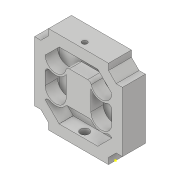
# Autodesk Inventor part: 20_Cube_Inser_Flexuremanipulator_zonly_translation_v3
Saved by Autodesk Inventor 2019.4 (Build 234330000, 330)
## iProperties
Created: 2019-07-01
Part Number: 20_Cube_Inser_Flexuremanipulator_zonly_translation_v3
Material: Generic
Document SubType Name: Modeling
Designer: diederichbenedict
Density: 1 g/cm^3
Appearance: Default
Author: diederichbenedict
Autodesk Inventor part; units mm, degrees
ref_plane "YZ Plane" through (0, 0, 0) normal (1, 0, 0) x (0, 1, 0)
ref_plane "XZ Plane" through (0, 0, 0) normal (0, 1, 0) x (-1, 0, 0)
ref_plane "Work Plane1" through (0, 0, 10) normal (0, 0, 1) x (1, 0, 0)
sketch "Sketch1" plane through (0, 0, 10) normal (0, 0, 1) x (1, 0, 0)
  line L0 (-4.0299, -0.3538) -> (-2.2322, 1.4439) construction
  arc A0 (-1.4439, 2.2322) -> (-2.2322, 1.4439) centre (-0.9299, 0.9299) ccw construction
  line L1 (-1.4439, 2.2322) -> (0.3538, 4.0299) construction
  line L2 (-37.8299, 42.8299) -> (-37.8299, 37.8299) construction
  line L3 (-37.8299, 37.8299) -> (-42.9208, 37.8299) construction
  line L4 (-37.8299, 42.2137) -> (-37.8299, 45.8299) construction
  line L5 (-37.8299, 45.8299) -> (-4.0299, 45.8299) construction
  line L6 (-4.0299, 45.8299) -> (-4.0299, 42.2137) construction
  line L7 (-4.0299, 4.0299) -> (0.3538, 4.0299) projected
  circle A1 centre (-20.9299, 20.9299) radius 17.5 projected
  line L8 (-20.9299, 58.9723) -> (17.1124, 20.9299) construction
  line L9 (17.1124, 20.9299) -> (-20.9299, -17.1124) construction
  line L10 (-20.9299, -17.1124) -> (-58.9723, 20.9299) construction
  line L11 (-58.9723, 20.9299) -> (-20.9299, 58.9723) construction
  line L12 (-20.9299, 58.9723) -> (-20.9299, -17.1124) construction
  line L13 (17.1124, 20.9299) -> (-58.9723, 20.9299) construction
  line L14 (-20.9299, 58.9723) -> (32.8701, 58.9723) construction
  line L15 (-43.4299, 43.4299) -> (1.5701, 43.4299) construction
  line L16 (1.5701, 43.4299) -> (1.5701, -1.5701) construction
  line L17 (1.5701, -1.5701) -> (-43.4299, -1.5701) construction
  line L18 (-43.4299, -1.5701) -> (-43.4299, 43.4299) construction
  line L19 (-43.4299, 43.4299) -> (1.5701, -1.5701) construction
  line L20 (1.5701, 43.4299) -> (-43.4299, -1.5701) construction
  line L21 (-43.4299, 5.3876) -> (-43.4299, 36.4723)
  line L22 (-43.4299, 36.4723) -> (-36.4723, 43.4299)
  line L23 (-36.4723, 43.4299) -> (-5.3876, 43.4299)
  line L24 (-5.3876, 43.4299) -> (1.5701, 36.4723)
  line L25 (1.5701, 36.4723) -> (1.5701, 5.3876)
  line L26 (1.5701, 5.3876) -> (-5.3876, -1.5701)
  line L27 (-5.3876, -1.5701) -> (-36.4723, -1.5701)
  line L28 (-36.4723, -1.5701) -> (-43.4299, 5.3876)
  line L29 (-4.0299, 42.2137) -> (-37.8299, 42.2137) projected
  line L30 (-4.0299, -0.3538) -> (-4.0299, 4.0299) projected
  circle A2 centre (-20.9299, 20.9299) radius 1.5
  line L31 (-10.9299, 10.9299) -> (-30.9299, 10.9299) construction
  line L32 (-30.9299, 10.9299) -> (-30.9299, 30.9299) construction
  line L33 (-30.9299, 30.9299) -> (-10.9299, 30.9299) construction
  line L34 (-10.9299, 30.9299) -> (-10.9299, 10.9299) construction
  line L35 (-10.9299, 10.9299) -> (-30.9299, 30.9299) construction
  line L36 (-30.9299, 10.9299) -> (-10.9299, 30.9299) construction
  circle A3 centre (-30.9299, 30.9299) radius 1.4
  circle A4 centre (-30.9299, 10.9299) radius 1.4
  circle A5 centre (-10.9299, 10.9299) radius 1.4
  line L37 (-45.8299, 37.8299) -> (-42.0723, 37.8299) construction
  line L38 (-42.1723, 37.7299) -> (-45.8299, 37.7299)
  line L39 (-45.8299, 37.7299) -> (-45.8299, 4.1299)
  line L40 (-45.8299, 4.1299) -> (-42.1723, 4.1299)
  line L41 (-42.1723, 4.1299) -> (-42.1723, 37.7299)
  line L42 (-45.8299, 4.0299) -> (-42.0723, 4.0299) construction
  line L43 (-45.8299, 37.8299) -> (-42.0723, 37.8299) projected
  line L44 (-37.7299, 45.8299) -> (-4.1299, 45.8299)
  line L45 (-4.1299, 45.8299) -> (-4.1299, 42.1723)
  line L46 (-4.1299, 42.1723) -> (-37.7299, 42.1723)
  line L47 (-37.7299, 42.1723) -> (-37.7299, 45.8299)
  line L48 (0.4701, 37.8299) -> (0.4701, 4.0299) construction
  line L49 (0.4701, 4.0299) -> (3.9701, 4.0299) construction
  line L50 (3.9701, 37.8299) -> (3.9701, 4.0299) construction
  line L51 (0.4701, 37.8299) -> (3.9701, 37.8299) construction
  line L52 (-45.8299, -3.9701) -> (-4.0299, -3.9701) construction
  line L53 (0.3124, 37.7299) -> (3.9701, 37.7299)
  line L54 (3.9701, 37.7299) -> (3.9701, 4.1299)
  line L55 (3.9701, 4.1299) -> (0.3124, 4.1299)
  line L56 (0.3124, 4.1299) -> (0.3124, 37.7299)
  line L57 (-4.1713, -0.3538) -> (-37.7299, -0.3538)
  line L58 (-37.7299, -0.3538) -> (-37.7299, -3.9701)
  line L59 (-37.7299, -3.9701) -> (-4.1713, -3.9701)
  line L60 (-4.1713, -3.9701) -> (-4.1713, -0.3538)
  point P0 (-37.8299, 4.0299)
  dimension "d18" = 53.8
  dimension "d19" = 45
  dimension "d20" = 53.8
  dimension "d21" = 45
  dimension "d22" = 45
  dimension "d30" = 20
  dimension "d31" = 20
  dimension "d32" = 2.8
  dimension "d33" = 2.8
  dimension "d34" = 2.8
  dimension "d35" = 3
  dimension "d36" = 0.1
  dimension "d37" = 0.1
  dimension "d38" = 0.1
  dimension "d39" = 0.1
  constraints: 86 end point, 21 point on line, 14 parallel, 8 perpendicular, 7 horizontal, 7 midpoint, 4 centre point, 4 coincident, 1 equal length
  measures "d18" distance of L8.start L8.end
  measures "d19" angle of L8 L14
  measures "d20" distance of L8.end L9.end
  measures "d21" distance of L16.end L17.end
  measures "d22" distance of L15.end L16.end
  measures "d30" distance of L32.end L33.end
  measures "d31" distance of L31.end L32.end
  measures "d32" diameter of A3
  measures "d33" diameter of A4
  measures "d34" diameter of A5
  measures "d35" diameter of A2
  measures "d36" distance between parallel lines of L38 L43
  measures "d37" distance between parallel lines of L40 L42
  measures "d38" distance between parallel lines of L45 L6
  measures "d39" distance between parallel lines of L4 L47
extrude "Extrusion1" add sketch "Sketch1" along normal blind 5 contours L30 L26 L57 L28 L41 L22 L46 L24 L56 L7 | L7 L26 L30 | L56 L24 L25 L26 | L26 L25 L24 L53 L54 L55 | L60 L59 L58 L57 L28 L27 L26 | L26 L27 L28 L57 | L46 L22 L29 L24 | L24 L29 L45 | L40 L39 L38 L22 L21 L28 | L28 L21 L22 L41 | L29 L22 L23 L24 | L24 L23 L22 L29 L47 L44 L45 | L47 L29 L22 | A1 | A2 | A3 | A4 | A5
sketch "Skizze4" plane through (0, 0, 15) normal (0, 0, 1) x (1, 0, 0)
  line L0 (-37.7299, 42.1723) -> (-42.1723, 37.7299) projected
  line L1 (-42.1723, 37.7299) -> (-45.8299, 37.7299) projected
  line L2 (-45.8299, 37.7299) -> (-45.8299, 4.1299) construction
  line L3 (-45.8299, 4.1299) -> (-42.1723, 4.1299) projected
  line L4 (-42.1723, 4.1299) -> (-37.6885, -0.3538) projected
  line L5 (-37.6885, -0.3538) -> (-37.7299, -0.3538) projected
  line L6 (-37.7299, -0.3538) -> (-37.7299, -3.9701) projected
  line L7 (-37.7299, -3.9701) -> (-4.1713, -3.9701) construction
  line L8 (-4.1713, -3.9701) -> (-4.1713, -0.3538) projected
  line L9 (-4.1713, -0.3538) -> (0.3124, 4.1299) projected
  line L10 (0.3124, 4.1299) -> (3.9701, 4.1299) projected
  line L11 (3.9701, 4.1299) -> (3.9701, 37.7299) construction
  line L12 (3.9701, 37.7299) -> (0.3124, 37.7299) projected
  line L13 (0.3124, 37.7299) -> (-4.1299, 42.1723) projected
  line L14 (-4.1299, 42.1723) -> (-4.1299, 45.8299) projected
  line L15 (-4.1299, 45.8299) -> (-37.7299, 45.8299) construction
  line L16 (-37.7299, 45.8299) -> (-37.7299, 42.1723) projected
  line L17 (-37.9299, 46.0299) -> (-3.9299, 46.0299) construction
  line L18 (-3.9299, 46.0299) -> (-3.9299, 42.2551)
  line L19 (-3.9299, 42.2551) -> (0.3953, 37.9299)
  line L20 (0.3953, 37.9299) -> (4.1701, 37.9299)
  line L21 (4.1701, 37.9299) -> (4.1701, 3.9299) construction
  line L22 (4.1701, 3.9299) -> (0.3953, 3.9299)
  line L23 (0.3953, 3.9299) -> (-3.9713, -0.4367)
  line L24 (-3.9713, -0.4367) -> (-3.9713, -4.1701)
  line L25 (-3.9713, -4.1701) -> (-37.9299, -4.1701) construction
  line L26 (-37.9299, -4.1701) -> (-37.9299, -0.3953)
  line L27 (-37.9299, -0.3953) -> (-42.2551, 3.9299)
  line L28 (-42.2551, 3.9299) -> (-46.0299, 3.9299)
  line L29 (-46.0299, 3.9299) -> (-46.0299, 37.9299) construction
  line L30 (-46.0299, 37.9299) -> (-42.2551, 37.9299)
  line L31 (-42.2551, 37.9299) -> (-37.9299, 42.2551)
  line L32 (-37.9299, 42.2551) -> (-37.9299, 46.0299)
  line L33 (-45.8299, 37.7299) -> (-45.8299, 37.9299)
  line L34 (-4.1299, 45.8299) -> (-37.7299, 45.8299) projected
  line L35 (-37.7299, 45.8299) -> (-37.9299, 45.8299)
  line L36 (-4.1299, 45.8299) -> (-3.9299, 45.8299)
  line L37 (3.9701, 37.7299) -> (3.9701, 37.9299)
  line L38 (3.9701, 4.1299) -> (3.9701, 37.7299) projected
  line L39 (3.9701, 4.1299) -> (3.9701, 3.9299)
  line L40 (-4.1713, -3.9701) -> (-3.9713, -3.9701)
  line L41 (-37.7299, -3.9701) -> (-37.9299, -3.9701)
  line L42 (-45.8299, 4.1299) -> (-45.8299, 3.9299)
  point P0 (0, 0)
  dimension "d40" = 0.2
  constraints: 48 end point, 12 point on line, 4 perpendicular, 15 other
  measures "d40" distance between parallel lines of L15 L17
extrude "IM_offset" add sketch "Skizze4" against normal up to surface (5 mm away)
sketch "Sketch5" plane through (0, 0, 15) normal (0, 0, 1) x (1, 0, 0)
  line L0 (-3.9299, 45.8299) -> (-37.9299, 45.8299) projected
  line L1 (-37.9299, 45.8299) -> (-37.9299, 42.2551) projected
  line L2 (-37.9299, 42.2551) -> (-42.2551, 37.9299) projected
  line L3 (-42.2551, 37.9299) -> (-45.8299, 37.9299) projected
  line L4 (-45.8299, 37.9299) -> (-45.8299, 3.9299) projected
  line L5 (-42.2551, 3.9299) -> (-45.8299, 3.9299) projected
  line L6 (-37.9299, -0.3953) -> (-42.2551, 3.9299) projected
  line L7 (-37.9299, -3.9701) -> (-37.9299, -0.3953) projected
  line L8 (-3.9713, -3.9701) -> (-37.9299, -3.9701) projected
  line L9 (-3.9713, -3.9701) -> (-3.9713, -0.4367) projected
  line L10 (-3.9713, -0.4367) -> (0.3953, 3.9299) projected
  line L11 (0.3953, 3.9299) -> (3.9701, 3.9299) projected
  line L12 (3.9701, 3.9299) -> (3.9701, 37.9299) projected
  line L13 (3.9701, 37.9299) -> (0.3953, 37.9299) projected
  line L14 (0.3953, 37.9299) -> (-3.9299, 42.2551) projected
  line L15 (-3.9299, 42.2551) -> (-3.9299, 45.8299) projected
  line L16 (-2.0299, 31.9299) -> (-2.0299, 9.9299)
  line L17 (-2.0299, 9.9299) -> (-2.09, 9.9299)
  line L18 (-2.09, 9.9299) -> (-9.9713, 2.0486)
  line L19 (-9.9713, 2.0486) -> (-9.9713, 2.0299)
  line L20 (-9.9713, 2.0299) -> (-31.9299, 2.0299)
  line L21 (-31.9299, 2.0299) -> (-31.9299, 2.09)
  line L22 (-31.9299, 2.09) -> (-39.7698, 9.9299)
  line L23 (-39.7698, 9.9299) -> (-39.8299, 9.9299)
  line L24 (-39.8299, 9.9299) -> (-39.8299, 31.9299)
  line L25 (-39.8299, 31.9299) -> (-39.7698, 31.9299)
  line L26 (-39.7698, 31.9299) -> (-31.9299, 39.7698)
  line L27 (-31.9299, 39.7698) -> (-31.9299, 39.8299)
  line L28 (-31.9299, 39.8299) -> (-9.9299, 39.8299)
  line L29 (-9.9299, 39.8299) -> (-9.9299, 39.7698)
  line L30 (-9.9299, 39.7698) -> (-2.09, 31.9299)
  line L31 (-2.09, 31.9299) -> (-2.0299, 31.9299)
  dimension "d46" = 6
  constraints: 32 end point, 15 other
  measures "d46" distance between parallel lines of L12 L16
extrude "Extrusion5" add sketch "Sketch5" along normal blind 8
sketch "Sketch6" plane through (0, 0, 23) normal (0, 0, 1) x (1, 0, 0)
  point P0 (0, 0)
sketch "Sketch7" plane through (0, 0, 23) normal (0, 0, 1) x (1, 0, 0)
  line L0 (-2.0299, 9.9299) -> (-2.09, 9.9299) projected
  line L1 (-2.09, 9.9299) -> (-9.9713, 2.0486) projected
  line L2 (-9.9713, 2.0486) -> (-9.9713, 2.0299) projected
  line L3 (-9.9713, 2.0299) -> (-31.9299, 2.0299) projected
  line L4 (-31.9299, 2.0299) -> (-31.9299, 2.09) projected
  line L5 (-31.9299, 2.09) -> (-39.7698, 9.9299) projected
  line L6 (-39.7698, 9.9299) -> (-39.8299, 9.9299) projected
  line L7 (-39.8299, 9.9299) -> (-39.8299, 31.9299) projected
  line L8 (-39.8299, 31.9299) -> (-39.7698, 31.9299) projected
  line L9 (-39.7698, 31.9299) -> (-31.9299, 39.7698) projected
  line L10 (-31.9299, 39.7698) -> (-31.9299, 39.8299) projected
  line L11 (-31.9299, 39.8299) -> (-9.9299, 39.8299) projected
  line L12 (-9.9299, 39.8299) -> (-9.9299, 39.7698) projected
  line L13 (-9.9299, 39.7698) -> (-2.09, 31.9299) projected
  line L14 (-2.09, 31.9299) -> (-2.0299, 31.9299) projected
  line L15 (-2.0299, 31.9299) -> (-2.0299, 9.9299) projected
  line L16 (-3.9299, 45.8299) -> (-37.9299, 45.8299) projected
  line L17 (-37.9299, 45.8299) -> (-37.9299, 42.2551) projected
  line L18 (-37.9299, 42.2551) -> (-42.2551, 37.9299) projected
  line L19 (-42.2551, 37.9299) -> (-45.8299, 37.9299) projected
  line L20 (-45.8299, 37.9299) -> (-45.8299, 3.9299) projected
  line L21 (-45.8299, 3.9299) -> (-42.2551, 3.9299) projected
  line L22 (-42.2551, 3.9299) -> (-37.9299, -0.3953) projected
  line L23 (-37.9299, -0.3953) -> (-37.9299, -3.9701) projected
  line L24 (-37.9299, -3.9701) -> (-3.9713, -3.9701) projected
  line L25 (-3.9713, -3.9701) -> (-3.9713, -0.4367) projected
  line L26 (-3.9713, -0.4367) -> (0.3953, 3.9299) projected
  line L27 (0.3953, 3.9299) -> (3.9701, 3.9299) projected
  line L28 (3.9701, 3.9299) -> (3.9701, 37.9299) projected
  line L29 (3.9701, 37.9299) -> (0.3953, 37.9299) projected
  line L30 (0.3953, 37.9299) -> (-3.9299, 42.2551) projected
  line L31 (-3.9299, 42.2551) -> (-3.9299, 45.8299) projected
  line L32 (-2.09, 9.9299) -> (-2.0299, 9.9299) projected
  line L33 (-2.0299, 9.9299) -> (-2.0299, 31.9299) projected
  line L34 (-2.0299, 31.9299) -> (-2.09, 31.9299) projected
  line L35 (-2.09, 31.9299) -> (-9.9299, 39.7698) projected
  line L36 (-9.9299, 39.7698) -> (-9.9299, 39.8299) projected
  line L37 (-9.9299, 39.8299) -> (-31.9299, 39.8299) projected
  line L38 (-31.9299, 39.8299) -> (-31.9299, 39.7698) projected
  line L39 (-31.9299, 39.7698) -> (-39.7698, 31.9299) projected
  line L40 (-39.7698, 31.9299) -> (-39.8299, 31.9299) projected
  line L41 (-39.8299, 31.9299) -> (-39.8299, 9.9299) projected
  line L42 (-39.8299, 9.9299) -> (-39.7698, 9.9299) projected
  line L43 (-39.7698, 9.9299) -> (-31.9299, 2.09) projected
  line L44 (-31.9299, 2.09) -> (-31.9299, 2.0299) projected
  line L45 (-31.9299, 2.0299) -> (-9.9713, 2.0299) projected
  line L46 (-9.9713, 2.0299) -> (-9.9713, 2.0486) projected
  line L47 (-9.9713, 2.0486) -> (-2.09, 9.9299) projected
  line L48 (-27.9299, 13.3383) -> (-20.9299, 13.3383)
  line L49 (-20.9299, 13.3383) -> (-20.9299, 31.9299)
  line L50 (-20.9299, 31.9299) -> (-27.9299, 31.9299)
  line L51 (-27.9299, 31.9299) -> (-27.9299, 13.3383)
  line L52 (-39.8299, 9.9299) -> (-39.8299, 31.9299) projected
  arc A0 (-39.8299, 31.9299) -> (-27.9299, 31.9299) centre (-33.8799, 31.93) ccw
  arc A1 (-39.8299, 28.3383) -> (-27.9299, 28.3383) centre (-33.8799, 31.93) ccw
  line L53 (-27.9299, 28.3383) -> (-39.8299, 28.3383) construction
  line L54 (-27.9299, 28.3383) -> (-16.0299, 28.3383) construction
  line L55 (-39.8299, 31.9299) -> (-39.8299, 28.3383)
  line L56 (-27.9299, 28.3383) -> (-27.9299, 31.9299)
  line L57 (-27.9299, 13.3383) -> (-27.9299, 16.9299)
  arc A2 (-39.8299, 13.3383) -> (-27.9299, 13.3383) centre (-33.8799, 16.93) ccw
  line L58 (-27.9299, 13.3383) -> (-39.8299, 13.3383) construction
  line L59 (-39.8299, 16.9299) -> (-39.8299, 13.3383)
  arc A3 (-39.8299, 16.9299) -> (-27.9299, 16.9299) centre (-33.8799, 16.93) ccw
  circle A4 centre (-20.9299, 20.9299) radius 18.9
  point P0 (0, 0)
  point P1 (-39.7698, 16.9299)
  point P2 (-39.7698, 16.9299)
  dimension "d51" = 0
  dimension "d52" = 180
  dimension "d55" = 15
  dimension "d60" = 0
  dimension "d61" = 1
  dimension "d63" = 0
  constraints: 22 end point, 10 point on circle, 5 centre point, 3 collinear, 3 point on line, 3 tangent, 2 concentric, 2 horizontal, 2 parallel, 1 perpendicular, 1 vertical, 15 other
  measures "d51" distance from line of L8.end L50
  measures "d52" angle of L53 L54
  measures "d55" distance of L7.end A3.start
  measures "d60" distance from line of L57.start L48
  measures "d61" radial gap between concentric circles of A0 A1
  measures "d63" distance from line of A4.centre L49
extrude "Extrusion6" add sketch "Sketch7" against normal blind 7 contours A4 A1 L7 A0 | A0 L51 A1 A4 | A4 A3 L51 A2 | A2 L7 A3 A4 | L50 L49 L48 L51
mirror "Mirror1" about plane through (-20.9299, 31.9299, 23) normal (1, 0, 0) of "Extrusion6"
fillet "Fillet1" radius 2 8 edges at (-27.9299, 13.3383, 19.5) (-13.9299, 13.3383, 19.5) (-13.9299, 31.9299, 19.5) (-27.9299, 31.9299, 19.5) (-2.0299, 28.3383, 19.5) (-2.0299, 13.3383, 19.5) (-39.8299, 28.3383, 19.5) (-39.8299, 13.3383, 19.5)
sketch "Sketch8" plane through (-37.9299, -3.9701, 10) normal (0, -1, 0) x (1, 0, 0)
  line L0 (22.9617, 13) -> (22.9617, 6) projected
  line L1 (11.0383, 13) -> (22.9617, 13) projected
  line L2 (11.0383, 6) -> (11.0383, 13) projected
  line L3 (11.0383, 6) -> (22.9617, 6) projected
  circle A0 centre (16.9793, 9.5) radius 2.45
  point P0 (37.9299, -10)
  dimension "d67" = 4.9
  constraints: 1 centre point
  measures "d67" diameter of A0
extrude "Extrusion7" cut sketch "Sketch8" against normal blind 7 contours A0
sketch "Sketch9" plane through (-37.9299, 45.8299, 10) normal (0, 1, 0) x (1, 0, 0)
  circle A0 centre (16.9793, -9.5) radius 2.45 projected
  circle A1 centre (16.9793, -9.5) radius 1.45
  point P0 (37.9299, 10)
  dimension "d70" = 2.9
  constraints: 1 centre point, 1 coincident
  measures "d70" diameter of A1
extrude "Extrusion8" cut sketch "Sketch9" against normal blind 7 contours A1
body "Solid1"
